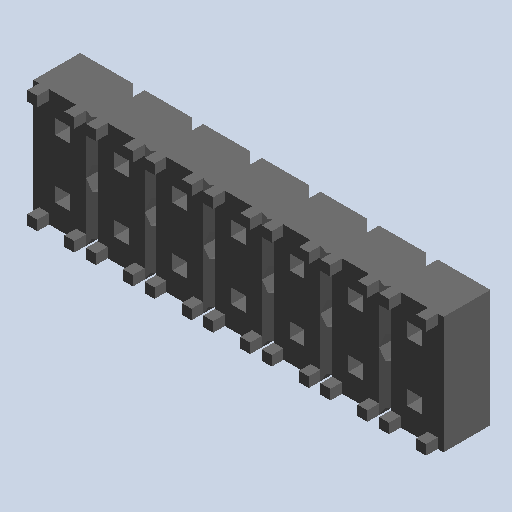
# Autodesk Inventor part: TSW-107-07-G-D_body
Saved by Autodesk Inventor 2024.2 (Build 282272000, 272)
## iProperties
Category: PARTsolutions
Company: SAMTEC
Part Number: TSW-107-07-G-D_body
Material: Generic
Catalog Web Link: www.cadenas.de
Description: TSW Series Body-TSW Series - (2,54 mm) .100" Through-Hole .025" Square Post Header
Vendor: SAMTEC
Document SubType Name: Modeling
Designer: partserver
Manufacturer: SAMTEC
Mass: 0.164867 g
Surface Area: 3.96379 cm^2
Volume: 0.164867 cm^3
Density: 1 g/cm^3
Appearance: PSOLRGB-127-127-127
PSOL_IDENT_0: {$CADENAS_DATA\23d-libs\samtec\modelling\tsw\parts\tsw_body.prj},234 {VTYP=3D},{NB=TSW-107-07-G-D_bo
PSOL_IDENT_1: dy},{LINA=TSW-107-07-G-D_body},{NN=TSW Series Body},{DATE=29.08.2019 09:17:37},{GEOMDATE=10.06.2019
PSOL_IDENT_2: 10:10:01},{VERSION=},{LINEID=10},{WBVAR=TSS,POS,LS,PLOPT,ROW,TOPT,LCOPT,LLOPT,POLOPT},{WBNUMERIC=POS
PSOL_IDENT_3: }  {NB=TSW-107-07-G-D_body},{LINA=TSW-107-07-G-D_body},{KT=DUMMY},{PN=TSW-107-07-G-D},{SERIES=TSW},{
PSOL_IDENT_4: TSS=-1},{POS=7},{POSALG=[1:50/1]},{POSPN=07},{BLS=0.7},{LS=-07},{LSALG= '-05','-05','-06','-06','-07'
PSOL_IDENT_5: ,'-07','-08','-08','-09','-09','-10','-10','-11','-11','-12','-12','-13','-13','-14','-14','-15','-1
PSOL_IDENT_6: 5','-16','-16','-17','-17','-18','-18','-19','-19','-20','-20','-21','-21','-22','-22','-23','-23','
PSOL_IDENT_7: -24','-24','-25','-25','-26','-26','-27','-27','-28','-28','-29','-29','-30','-30' },{PLOPT=-G},{PLO
PSOL_IDENT_8: PTALG= '-G','-G - 10micro\" Gold in Contact Area, 3micro\" Gold on Tail','-T','-T - Matte Tin Contac
PSOL_IDENT_9: t and Tail','-S','-S - 30micro\" Selective Gold in Contact Area, Matte Tin on Tail','-H','-H - 30mic
PSOL_IDENT_10: ro\" Heavy Gold in Contact Area, 3micro\" Gold on Tail','-L','-L - 10micro\" Light Selective Gold in
PSOL_IDENT_11: Contact Area, Matte Tin on Tail','-F','-F - 3micro\" Flash Selective Gold in Contact Area, Matte Ti
PSOL_IDENT_12: n on Tail','-E','-E - 50micro\" Extra Heavy Gold in Contact Area, 3micro\" Gold on Tail','-TL','-TL
PSOL_IDENT_13: - Tin/Lead (90/10 +/-5%) Contact and Tail','-TM','-TM - Matte Tin Contact and Tail','-SM','-SM - 30m
PSOL_IDENT_14: icro\" Selective Gold in Contact Area, Matte Tin on Tail','-LM','-LM - 10micro\" Light Selective Gol
PSOL_IDENT_15: d in Contact Area, Matte Tin on Tail','-FM','-FM - 3micro\" Flash Selective Gold in Contact Area, Ma
PSOL_IDENT_16: tte Tin on Tail','-SS','-SS - 30micro\" Stripe Selective Gold in Contact Area, Matte Tin on Tail' },
PSOL_IDENT_17: {ROW=-D},{ROWALG= '-S','-S - Single','-D','-D - Double','-T','-T - Triple','-Q','-Q - Triple (Fill O
PSOL_IDENT_18: uter Rows only)' },{TOPT=},{TOPTALG= '','Straight Body' },{ST= '','Straight Body' },{RA=},{RE=},{NA=
PSOL_IDENT_19: },{NE=},{LA=},{LCOPT=},{LCOPTALG= '','Not Available' },{LLOPT=},{LLOPTALG= '','Not Selected','-LL','
PSOL_IDENT_20: -LL - Locking Lead' },{POLOPT=},{POLOPTALG= '','Not Selected','001','001','002','002','003','003','0
PSOL_IDENT_21: 04','004','005','005','006','006','007','007','008','008','009','009','010','010','011','011','012','
PSOL_IDENT_22: 012','013','013','014','014' },{POLOPTMAX=168},{POLOPTMAX2='001','001','002','002','003','003','004'
PSOL_IDENT_23: ,'004','005','005','006','006','007','007','008','008','009','009','010','010','011','011','012','01
PSOL_IDENT_24: 2','013','013','014','014'},{POLARIZE='001','001','002','002','003','003','004','004','005','005','0
PSOL_IDENT_25: 06','006','007','007','008','008','009','009','010','010','011','011','012','012','013','013','014','
PSOL_IDENT_26: 014','015','015','016','016','017','017','018','018','019','019','020','020','021','021','022','022'
PSOL_IDENT_27: ,'023','023','024','024','025','025','026','026','027','027','028','028','029','029','030','030','03
PSOL_IDENT_28: 1','031','032','032','033','033','034','034','035','035','036','036','037','037','038','038','039','
PSOL_IDENT_29: 039','040','040','041','041','042','042','043','043','044','044','045','045','046','046','047','047'
PSOL_IDENT_30: ,'048','048','049','049','050','050','051','051','052','052','053','053','054','054','055','055','05
PSOL_IDENT_31: 6','056','057','057','058','058','059','059','060','060','061','061','062','062','063','063','064','
PSOL_IDENT_32: 064','065','065','066','066','067','067','068','068','069','069','070','070','071','071','072','072'
PSOL_IDENT_33: ,'073','073','074','074','075','075','076','076','077','077','078','078','079','079','080','080','08
PSOL_IDENT_34: 1','081','082','082','083','083','084','084','085','085','086','086','087','087','088','088','089','
PSOL_IDENT_35: 089','090','090','091','091','092','092','093','093','094','094','095','095','096','096','097','097'
PSOL_IDENT_36: ,'098','098','099','099','100','100','101','101','102','102','103','103','104','104','105','105','10
PSOL_IDENT_37: 6','106','107','107','108','108','109','109','110','110','111','111','112','112','113','113','114','
PSOL_IDENT_38: 114','115','115','116','116','117','117','118','118','119','119','120','120','121','121','122','122'
PSOL_IDENT_39: ,'123','123','124','124','125','125','126','126','127','127','128','128','129','129','130','130','13
PSOL_IDENT_40: 1','131','132','132','133','133','134','134','135','135','136','136','137','137','138','138','139','
PSOL_IDENT_41: 139','140','140','141','141','142','142','143','143','144','144','145','145','146','146','147','147'
PSOL_IDENT_42: ,'148','148','149','149','150','150'},{POLOPTPN=},{A=0.700},{E=0.000},{C=0.230},{BW=0.200},{SM=1},{F=
PSOL_IDENT_43: 0.910},{G=0.198},{PP=0.00000}
NB: TSW-107-07-G-D_body
NN: TSW Series Body
NT: TSW Series - (2,54 mm) .100" Through-Hole .025" Square Post Header
NBSYN: $PN._body
LINA: TSW-107-07-G-D_body
CATALOG: Samtec
SERIES: TSW
TSS: -1 - .100 [2.54] Fill every position
POS: 7
LS: -07
PLOPT: -G - 10micro" Gold in Contact Area, 3micro" Gold on Tail
ROW: -D - Double
TOPT: Straight Body
LCOPT: Not Available
LLOPT: Not Selected
POLOPT: Not Selected
SUPPLIER: SAMTEC
ARTICLENO: TSW-107-07-G-D_body
BOMINFO: TSW-107-07-G-D_body
CREATOR: CADENAS GmbH
Title: TSW-107-07-G-D_body
Author: Cadenas PARTsolutions
Comments: TSW Series - (2,54 mm) .100" Through-Hole .025" Square Post Header
Autodesk Inventor part; units mm, degrees
sketch "Sketch_1" plane through (0, 0, 0) normal (0, 1, 0) x (-1, 0, 0)
  line L0 (8.89, -2.54) -> (8.89, 2.54)
  line L1 (8.89, 2.54) -> (-8.89, 2.54)
  line L2 (-8.89, 2.54) -> (-8.89, -2.54)
  line L3 (-8.89, -2.54) -> (8.89, -2.54)
  line L4 (-7.3025, 0.9525) -> (-7.3025, 1.5875)
  line L5 (-7.3025, 1.5875) -> (-7.9375, 1.5875)
  line L6 (-7.9375, 1.5875) -> (-7.9375, 0.9525)
  line L7 (-7.9375, 0.9525) -> (-7.3025, 0.9525)
  line L8 (-7.3025, -1.5875) -> (-7.3025, -0.9525)
  line L9 (-7.3025, -0.9525) -> (-7.9375, -0.9525)
  line L10 (-7.9375, -0.9525) -> (-7.9375, -1.5875)
  line L11 (-7.9375, -1.5875) -> (-7.3025, -1.5875)
  line L12 (-4.7625, 0.9525) -> (-4.7625, 1.5875)
  line L13 (-4.7625, 1.5875) -> (-5.3975, 1.5875)
  line L14 (-5.3975, 1.5875) -> (-5.3975, 0.9525)
  line L15 (-5.3975, 0.9525) -> (-4.7625, 0.9525)
  line L16 (-4.7625, -1.5875) -> (-4.7625, -0.9525)
  line L17 (-4.7625, -0.9525) -> (-5.3975, -0.9525)
  line L18 (-5.3975, -0.9525) -> (-5.3975, -1.5875)
  line L19 (-5.3975, -1.5875) -> (-4.7625, -1.5875)
  line L20 (-2.2225, 0.9525) -> (-2.2225, 1.5875)
  line L21 (-2.2225, 1.5875) -> (-2.8575, 1.5875)
  line L22 (-2.8575, 1.5875) -> (-2.8575, 0.9525)
  line L23 (-2.8575, 0.9525) -> (-2.2225, 0.9525)
  line L24 (-2.2225, -1.5875) -> (-2.2225, -0.9525)
  line L25 (-2.2225, -0.9525) -> (-2.8575, -0.9525)
  line L26 (-2.8575, -0.9525) -> (-2.8575, -1.5875)
  line L27 (-2.8575, -1.5875) -> (-2.2225, -1.5875)
  line L28 (0.3175, 0.9525) -> (0.3175, 1.5875)
  line L29 (0.3175, 1.5875) -> (-0.3175, 1.5875)
  line L30 (-0.3175, 1.5875) -> (-0.3175, 0.9525)
  line L31 (-0.3175, 0.9525) -> (0.3175, 0.9525)
  line L32 (0.3175, -1.5875) -> (0.3175, -0.9525)
  line L33 (0.3175, -0.9525) -> (-0.3175, -0.9525)
  line L34 (-0.3175, -0.9525) -> (-0.3175, -1.5875)
  line L35 (-0.3175, -1.5875) -> (0.3175, -1.5875)
  line L36 (2.8575, 0.9525) -> (2.8575, 1.5875)
  line L37 (2.8575, 1.5875) -> (2.2225, 1.5875)
  line L38 (2.2225, 1.5875) -> (2.2225, 0.9525)
  line L39 (2.2225, 0.9525) -> (2.8575, 0.9525)
  line L40 (2.8575, -1.5875) -> (2.8575, -0.9525)
  line L41 (2.8575, -0.9525) -> (2.2225, -0.9525)
  line L42 (2.2225, -0.9525) -> (2.2225, -1.5875)
  line L43 (2.2225, -1.5875) -> (2.8575, -1.5875)
  line L44 (5.3975, 0.9525) -> (5.3975, 1.5875)
  line L45 (5.3975, 1.5875) -> (4.7625, 1.5875)
  line L46 (4.7625, 1.5875) -> (4.7625, 0.9525)
  line L47 (4.7625, 0.9525) -> (5.3975, 0.9525)
  line L48 (5.3975, -1.5875) -> (5.3975, -0.9525)
  line L49 (5.3975, -0.9525) -> (4.7625, -0.9525)
  line L50 (4.7625, -0.9525) -> (4.7625, -1.5875)
  line L51 (4.7625, -1.5875) -> (5.3975, -1.5875)
  line L52 (7.9375, 0.9525) -> (7.9375, 1.5875)
  line L53 (7.9375, 1.5875) -> (7.3025, 1.5875)
  line L54 (7.3025, 1.5875) -> (7.3025, 0.9525)
  line L55 (7.3025, 0.9525) -> (7.9375, 0.9525)
  line L56 (7.9375, -1.5875) -> (7.9375, -0.9525)
  line L57 (7.9375, -0.9525) -> (7.3025, -0.9525)
  line L58 (7.3025, -0.9525) -> (7.3025, -1.5875)
  line L59 (7.3025, -1.5875) -> (7.9375, -1.5875)
  constraints: 120 end point
extrude "Extrusion1" add sketch "Sketch_1" along normal blind 2.54
sketch "Sketch_2" plane through (0, 0, 0) normal (0, 0, 1) x (1, 0, 0)
  line L0 (-6.604, 2.54) -> (-6.35, 2.286)
  line L1 (-6.35, 2.286) -> (-6.096, 2.54)
  line L2 (-6.096, 2.54) -> (-4.064, 2.54)
  line L3 (-4.064, 2.54) -> (-3.81, 2.286)
  line L4 (-3.81, 2.286) -> (-3.556, 2.54)
  line L5 (-3.556, 2.54) -> (-1.524, 2.54)
  line L6 (-1.524, 2.54) -> (-1.27, 2.286)
  line L7 (-1.27, 2.286) -> (-1.016, 2.54)
  line L8 (-1.016, 2.54) -> (1.016, 2.54)
  line L9 (1.016, 2.54) -> (1.27, 2.286)
  line L10 (1.27, 2.286) -> (1.524, 2.54)
  line L11 (1.524, 2.54) -> (3.556, 2.54)
  line L12 (3.556, 2.54) -> (3.81, 2.286)
  line L13 (3.81, 2.286) -> (4.064, 2.54)
  line L14 (4.064, 2.54) -> (6.096, 2.54)
  line L15 (6.096, 2.54) -> (6.35, 2.286)
  line L16 (6.35, 2.286) -> (6.604, 2.54)
  line L17 (6.604, 2.54) -> (6.604, 3.556)
  line L18 (6.604, 3.556) -> (-6.604, 3.556)
  line L19 (-6.604, 3.556) -> (-6.604, 2.54)
  constraints: 40 end point
extrude "Extrusion2" cut sketch "Sketch_2" along normal mid plane 35.56
sketch "Sketch_3" plane through (0, 0, 0) normal (0, 0, 1) x (1, 0, 0)
  line L0 (-6.604, 0.508) -> (-6.604, -0.508)
  line L1 (-6.604, -0.508) -> (6.604, -0.508)
  line L2 (6.604, -0.508) -> (6.604, 0.508)
  line L3 (6.604, 0.508) -> (6.35, 0.762)
  line L4 (6.35, 0.762) -> (6.096, 0.508)
  line L5 (6.096, 0.508) -> (6.096, 0)
  line L6 (6.096, 0) -> (4.064, 0)
  line L7 (4.064, 0) -> (4.064, 0.508)
  line L8 (4.064, 0.508) -> (3.81, 0.762)
  line L9 (3.81, 0.762) -> (3.556, 0.508)
  line L10 (3.556, 0.508) -> (3.556, 0)
  line L11 (3.556, 0) -> (1.524, 0)
  line L12 (1.524, 0) -> (1.524, 0.508)
  line L13 (1.524, 0.508) -> (1.27, 0.762)
  line L14 (1.27, 0.762) -> (1.016, 0.508)
  line L15 (1.016, 0.508) -> (1.016, 0)
  line L16 (1.016, 0) -> (-1.016, 0)
  line L17 (-1.016, 0) -> (-1.016, 0.508)
  line L18 (-1.016, 0.508) -> (-1.27, 0.762)
  line L19 (-1.27, 0.762) -> (-1.524, 0.508)
  line L20 (-1.524, 0.508) -> (-1.524, 0)
  line L21 (-1.524, 0) -> (-3.556, 0)
  line L22 (-3.556, 0) -> (-3.556, 0.508)
  line L23 (-3.556, 0.508) -> (-3.81, 0.762)
  line L24 (-3.81, 0.762) -> (-4.064, 0.508)
  line L25 (-4.064, 0.508) -> (-4.064, 0)
  line L26 (-4.064, 0) -> (-6.096, 0)
  line L27 (-6.096, 0) -> (-6.096, 0.508)
  line L28 (-6.096, 0.508) -> (-6.35, 0.762)
  line L29 (-6.35, 0.762) -> (-6.604, 0.508)
  constraints: 60 end point
extrude "Extrusion3" cut sketch "Sketch_3" along normal mid plane 35.56
sketch "Sketch_6" plane through (0, 0, 0) normal (0, 0, 1) x (1, 0, 0)
  line L0 (-9.8137, -0.254) -> (9.8137, -0.254)
  line L1 (9.8137, -0.254) -> (9.8137, 0.508)
  line L2 (9.8137, 0.508) -> (8.6391, 0.508)
  line L3 (8.6391, 0.508) -> (8.6391, 0)
  line L4 (8.6391, 0) -> (-8.6391, 0)
  line L5 (-8.6391, 0) -> (-8.6391, 0.508)
  line L6 (-8.6391, 0.508) -> (-9.8137, 0.508)
  line L7 (-9.8137, 0.508) -> (-9.8137, -0.254)
  constraints: 16 end point
extrude "Extrusion4" cut sketch "Sketch_6" along normal mid plane 10.16
sketch "Sketch_9" plane through (0, 0, 0) normal (0, 0, 1) x (1, 0, 0)
  line L0 (-8.2073, -0.254) -> (8.2073, -0.254)
  line L1 (8.2073, -0.254) -> (8.2073, 0.508)
  line L2 (8.2073, 0.508) -> (7.0327, 0.508)
  line L3 (7.0327, 0.508) -> (7.0327, 0)
  line L4 (7.0327, 0) -> (5.6673, 0)
  line L5 (5.6673, 0) -> (5.6673, 0.508)
  line L6 (5.6673, 0.508) -> (4.4927, 0.508)
  line L7 (4.4927, 0.508) -> (4.4927, 0)
  line L8 (4.4927, 0) -> (3.1273, 0)
  line L9 (3.1273, 0) -> (3.1273, 0.508)
  line L10 (3.1273, 0.508) -> (1.9527, 0.508)
  line L11 (1.9527, 0.508) -> (1.9527, 0)
  line L12 (1.9527, 0) -> (0.5873, 0)
  line L13 (0.5873, 0) -> (0.5873, 0.508)
  line L14 (0.5873, 0.508) -> (-0.5873, 0.508)
  line L15 (-0.5873, 0.508) -> (-0.5873, 0)
  line L16 (-0.5873, 0) -> (-1.9527, 0)
  line L17 (-1.9527, 0) -> (-1.9527, 0.508)
  line L18 (-1.9527, 0.508) -> (-3.1273, 0.508)
  line L19 (-3.1273, 0.508) -> (-3.1273, 0)
  line L20 (-3.1273, 0) -> (-4.4927, 0)
  line L21 (-4.4927, 0) -> (-4.4927, 0.508)
  line L22 (-4.4927, 0.508) -> (-5.6673, 0.508)
  line L23 (-5.6673, 0.508) -> (-5.6673, 0)
  line L24 (-5.6673, 0) -> (-7.0327, 0)
  line L25 (-7.0327, 0) -> (-7.0327, 0.508)
  line L26 (-7.0327, 0.508) -> (-8.2073, 0.508)
  line L27 (-8.2073, 0.508) -> (-8.2073, -0.254)
  constraints: 56 end point
extrude "Extrusion5" cut sketch "Sketch_9" along normal mid plane 10.16
sketch "Sketch_11" plane through (0, 0, 0) normal (1, 0, 0) x (0, 1, 0)
  line L0 (-0.254, 2.1082) -> (-0.254, -2.1082)
  line L1 (-0.254, -2.1082) -> (0.508, -2.1082)
  line L2 (0.508, -2.1082) -> (0.508, 2.1082)
  line L3 (0.508, 2.1082) -> (-0.254, 2.1082)
  constraints: 8 end point
extrude "Extrusion6" cut sketch "Sketch_11" along normal mid plane 35.56
sketch "Sketch_18" plane through (0, 0, 0) normal (0, 1, 0) x (-1, 0, 0)
  line L0 (6.604, -2.54) -> (6.4801, -2.286)
  line L1 (6.4801, -2.286) -> (6.2199, -2.286)
  line L2 (6.2199, -2.286) -> (6.096, -2.54)
  line L3 (6.096, -2.54) -> (4.064, -2.54)
  line L4 (4.064, -2.54) -> (3.9401, -2.286)
  line L5 (3.9401, -2.286) -> (3.6799, -2.286)
  line L6 (3.6799, -2.286) -> (3.556, -2.54)
  line L7 (3.556, -2.54) -> (1.524, -2.54)
  line L8 (1.524, -2.54) -> (1.4001, -2.286)
  line L9 (1.4001, -2.286) -> (1.1399, -2.286)
  line L10 (1.1399, -2.286) -> (1.016, -2.54)
  line L11 (1.016, -2.54) -> (-1.016, -2.54)
  line L12 (-1.016, -2.54) -> (-1.1399, -2.286)
  line L13 (-1.1399, -2.286) -> (-1.4001, -2.286)
  line L14 (-1.4001, -2.286) -> (-1.524, -2.54)
  line L15 (-1.524, -2.54) -> (-3.556, -2.54)
  line L16 (-3.556, -2.54) -> (-3.6799, -2.286)
  line L17 (-3.6799, -2.286) -> (-3.9401, -2.286)
  line L18 (-3.9401, -2.286) -> (-4.064, -2.54)
  line L19 (-4.064, -2.54) -> (-6.096, -2.54)
  line L20 (-6.096, -2.54) -> (-6.2199, -2.286)
  line L21 (-6.2199, -2.286) -> (-6.4801, -2.286)
  line L22 (-6.4801, -2.286) -> (-6.604, -2.54)
  line L23 (-6.604, -2.54) -> (-6.604, -3.048)
  line L24 (-6.604, -3.048) -> (6.604, -3.048)
  line L25 (6.604, -3.048) -> (6.604, -2.54)
  constraints: 52 end point
extrude "Extrusion7" cut sketch "Sketch_18" along normal mid plane 10.16
sketch "Sketch_20" plane through (0, 0, 0) normal (0, 1, 0) x (-1, 0, 0)
  line L0 (6.604, 2.54) -> (6.604, 4.826)
  line L1 (6.604, 4.826) -> (-6.604, 4.826)
  line L2 (-6.604, 4.826) -> (-6.604, 2.54)
  line L3 (-6.604, 2.54) -> (-6.4801, 2.286)
  line L4 (-6.4801, 2.286) -> (-6.2199, 2.286)
  line L5 (-6.2199, 2.286) -> (-6.096, 2.54)
  line L6 (-6.096, 2.54) -> (-6.096, 3.048)
  line L7 (-6.096, 3.048) -> (-4.064, 3.048)
  line L8 (-4.064, 3.048) -> (-4.064, 2.54)
  line L9 (-4.064, 2.54) -> (-3.9401, 2.286)
  line L10 (-3.9401, 2.286) -> (-3.6799, 2.286)
  line L11 (-3.6799, 2.286) -> (-3.556, 2.54)
  line L12 (-3.556, 2.54) -> (-3.556, 3.048)
  line L13 (-3.556, 3.048) -> (-1.524, 3.048)
  line L14 (-1.524, 3.048) -> (-1.524, 2.54)
  line L15 (-1.524, 2.54) -> (-1.4001, 2.286)
  line L16 (-1.4001, 2.286) -> (-1.1399, 2.286)
  line L17 (-1.1399, 2.286) -> (-1.016, 2.54)
  line L18 (-1.016, 2.54) -> (-1.016, 3.048)
  line L19 (-1.016, 3.048) -> (1.016, 3.048)
  line L20 (1.016, 3.048) -> (1.016, 2.54)
  line L21 (1.016, 2.54) -> (1.1399, 2.286)
  line L22 (1.1399, 2.286) -> (1.4001, 2.286)
  line L23 (1.4001, 2.286) -> (1.524, 2.54)
  line L24 (1.524, 2.54) -> (1.524, 3.048)
  line L25 (1.524, 3.048) -> (3.556, 3.048)
  line L26 (3.556, 3.048) -> (3.556, 2.54)
  line L27 (3.556, 2.54) -> (3.6799, 2.286)
  line L28 (3.6799, 2.286) -> (3.9401, 2.286)
  line L29 (3.9401, 2.286) -> (4.064, 2.54)
  line L30 (4.064, 2.54) -> (4.064, 3.048)
  line L31 (4.064, 3.048) -> (6.096, 3.048)
  line L32 (6.096, 3.048) -> (6.096, 2.54)
  line L33 (6.096, 2.54) -> (6.2199, 2.286)
  line L34 (6.2199, 2.286) -> (6.4801, 2.286)
  line L35 (6.4801, 2.286) -> (6.604, 2.54)
  constraints: 72 end point
extrude "Extrusion8" cut sketch "Sketch_20" along normal mid plane 10.16
sketch "Sketch_17" plane through (0, 0, 0) normal (0, 1, 0) x (-1, 0, 0)
  line L0 (6.604, 0) -> (6.4668, 0.508)
  line L1 (6.4668, 0.508) -> (6.2332, 0.508)
  line L2 (6.2332, 0.508) -> (6.096, 0)
  line L3 (6.096, 0) -> (6.2332, -0.508)
  line L4 (6.2332, -0.508) -> (6.4668, -0.508)
  line L5 (6.4668, -0.508) -> (6.604, 0)
  constraints: 12 end point
extrude "Extrusion9" cut sketch "Sketch_17" along normal mid plane 5.08
pattern_linear "Rectangular Pattern1" count 6 spacing 2.54 along (1, 0, 0) of "Extrusion9"
ref_plane "body_XY" through (0, 0, 0) normal (0, 1, 0) x (1, 0, 0)
ref_plane "body_YZ" through (0, 0, 0) normal (1, 0, 0) x (0, 0, -1)
ref_plane "body_ZX" through (0, 0, 0) normal (0, 0, -1) x (0, 1, 0)
ref_plane "pin_XY" through (0, 0, 0) normal (0, 1, 0) x (1, 0, 0)
ref_plane "pin_YZ" through (0, 0, 0) normal (1, 0, 0) x (0, 0, -1)
ref_plane "pin_ZX" through (0, 0, 0) normal (0, 0, -1) x (0, 1, 0)
body "Solid1"
